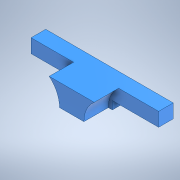
# Autodesk Inventor part: HullMid
Saved by Autodesk Inventor 2021 (Build 250183000, 183)
## iProperties
Created: 2021-05-14
Part Number: HullMid
Material: Generic
Document SubType Name: Modeling
Designer: ermoz
Density: 1 g/cm^3
Appearance: Default
Author: ermoz
Autodesk Inventor part; units mm, degrees
ref_plane "YZ Plane" through (0, 0, 0) normal (1, 0, 0) x (0, 1, 0)
ref_plane "XZ Plane" through (0, 0, 0) normal (0, 1, 0) x (-1, 0, 0)
ref_plane "XY Plane" through (0, 0, 0) normal (0, 0, 1) x (1, 0, 0)
sketch "Sketch1" plane through (0, 0, 0) normal (0, 1, 0) x (-1, 0, 0)
  line L0 (0, 0) -> (78.5, 0)
  line L1 (78.5, 0) -> (78.5, -9)
  line L2 (78.5, -9) -> (0, -9)
  line L3 (0, -9) -> (0, 0)
  line L4 (50.291, 0) -> (28.6614, 0)
  line L5 (78.5, -9) -> (69.5, -9)
  line L6 (69.5, -9) -> (69.5, 0)
  line L7 (69.5, 0) -> (78.5, 0)
  line L8 (78.5, 0) -> (78.5, -9)
  line L9 (69.5, -9) -> (57.5, -9)
  line L10 (57.5, -9) -> (57.5, 0)
  line L11 (57.5, 0) -> (69.5, 0)
  line L12 (69.5, 0) -> (69.5, -9)
  line L13 (19.5, -9) -> (7.5, -9)
  line L14 (7.5, -9) -> (7.5, 0)
  line L15 (7.5, 0) -> (19.5, 0)
  line L16 (19.5, 0) -> (19.5, -9)
  line L17 (69.5, -9) -> (57.5, -9)
  line L18 (19.5, -9) -> (7.5, -9)
  line L19 (69.5, -9) -> (57.5, -9)
  line L20 (57.5, -9) -> (57.5, 0)
  line L21 (57.5, 0) -> (69.5, 0)
  line L22 (69.5, 0) -> (69.5, -9)
  line L23 (69.5, -9) -> (57.5, 0) construction
  line L24 (57.5, -9) -> (69.5, 0) construction
  line L25 (7.5, -9) -> (19.5, -9)
  line L26 (19.5, -9) -> (19.5, 0)
  line L27 (19.5, 0) -> (7.5, 0)
  line L28 (7.5, 0) -> (7.5, -9)
  line L29 (7.5, -9) -> (19.5, 0) construction
  line L30 (19.5, -9) -> (7.5, 0) construction
  line L31 (63.5, 0) -> (13.5, 0)
  line L32 (13.5, 0) -> (13.5, 15)
  line L33 (13.5, 15) -> (63.5, 15)
  line L34 (63.5, 15) -> (63.5, 0)
  point P0 (63.5, -4.5)
  point P1 (13.5, -4.5)
  point P2 (13.5, 0)
  dimension "d0" = 78.5
  dimension "d1" = 9
  dimension "d3" = 9
  dimension "d4" = 12
  dimension "d5" = 12
  dimension "d6" = 50
  dimension "d7" = 15
  constraints: 70 end point, 14 parallel, 8 horizontal, 7 perpendicular, 5 midpoint, 4 point on line, 2 collinear
  measures "d0" distance of L1.end L2.end
  measures "d1" distance of L0.end L1.end
  measures "d3" distance of L6.end L7.end
  measures "d4" distance of L10.end L11.end
  measures "d5" distance of L14.end L15.end
  measures "d6" distance of point (13.5, -4.5) point (63.5, -4.5)
  measures "d7" distance of L31.end L32.end
extrude "Extrusion1" add sketch "Sketch1" along normal blind 13.5
sketch "Sketch2" plane through (-63.5, 0, 15) normal (0, 0, 1) x (1, 0, 0)
  line L0 (0, 0) -> (0, 13.5) projected
  circle A0 centre (0, 0) radius 15.5
  line L1 (50, 0) -> (50, 13.5) projected
  circle A1 centre (50, 0) radius 15.5
  circle A2 centre (0, 0) radius 17.5
  circle A3 centre (50, 0) radius 17.5
  line L2 (6, -5) -> (-6, -5)
  line L3 (-6, -5) -> (-6, 5)
  line L4 (-6, 5) -> (6, 5)
  line L5 (6, 5) -> (6, -5)
  line L6 (6, -5) -> (-6, 5) construction
  line L7 (-6, -5) -> (6, 5) construction
  line L8 (56, -5) -> (44, -5)
  line L9 (44, -5) -> (44, 5)
  line L10 (44, 5) -> (56, 5)
  line L11 (56, 5) -> (56, -5)
  line L12 (56, -5) -> (44, 5) construction
  line L13 (44, -5) -> (56, 5) construction
  line L14 (56, 5) -> (73.1985, 5)
  line L15 (63.5, 0) -> (63.5, 13.5) projected
  line L16 (44, 5) -> (35, 5)
  line L17 (35, 5) -> (35, 0)
  line L18 (35, 0) -> (15, 0)
  line L19 (63.5, 0) -> (-15, 0) projected
  line L20 (15, 5) -> (6, 5)
  line L21 (15, 5) -> (15, 0)
  line L22 (-6, 5) -> (-20.1894, 5)
  point P0 (-16.7705, 5)
  point P1 (17.5, 0)
  point P2 (6, 0)
  point P3 (-6, 0)
  point P4 (63.5, 5)
  dimension "d10" = 31
  dimension "d11" = 31
  dimension "d12" = 2
  dimension "d13" = 2
  dimension "d14" = 12
  dimension "d15" = 10
  dimension "d16" = 12
  dimension "d17" = 10
  dimension "d18" = 9
  dimension "d19" = 9
  constraints: 38 end point, 5 parallel, 5 perpendicular, 4 centre point, 4 horizontal, 4 midpoint, 2 point on line
  measures "d10" diameter of A0
  measures "d11" diameter of A1
  measures "d12" radial gap between concentric circles of A0 A2
  measures "d13" radial gap between concentric circles of A1 A3
  measures "d14" distance of L3.end L4.end
  measures "d15" distance of L2.end L3.end
  measures "d16" distance of L9.end L10.end
  measures "d17" distance of L8.end L9.end
  measures "d18" distance of L20.start L4.end
  measures "d19" distance of L9.end L16.end
extrude "Extrusion2" cut sketch "Sketch2" against normal up to surface (15 mm away)
extrude "Extrusion3" cut sketch "Sketch2" against normal through all contours L19 L3 L4 L0 | L0 L4 L5 L19 | L19 L18 A0 L22 L3 L2 L5 | L5 L20 A0 L21 L19 | A0 L18 A2 L22 | L20 L21 A0 | L19 L9 L10 L1 | L1 L10 L11 L19 | L11 L14 L15 L19 | L19 L17 A1 L16 L9 | A1 L17 L16
sketch "Sketch3" plane through (0, 13.5, -9) normal (0, 0, -1) x (-1, 0, 0)
  line L0 (28.5, -8.5) -> (28.5, -13.5) projected
  line L1 (48.5, -8.5) -> (48.5, -13.5) projected
  line L2 (28.5, -8.5) -> (48.5, -8.5)
  line L3 (48.5, -8.5) -> (48.5, -13.5)
  line L4 (48.5, -13.5) -> (28.5, -13.5)
  line L5 (28.5, -13.5) -> (28.5, -8.5)
  point P0 (0, -13.5)
  constraints: 8 end point, 2 parallel, 1 horizontal, 1 perpendicular
extrude "Extrusion4" cut sketch "Sketch3" against normal blind 4
body "Solid1"
